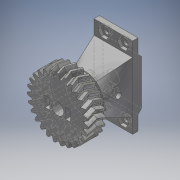
# Autodesk Inventor part: Swivel Joint Driven
Saved by Autodesk Inventor 2019 (Build 230136000, 136)
## iProperties
Created: 2020-04-05
Part Number: Swivel Joint Driven
Material: Steel
Document SubType Name: Modeling
Designer: isaac
Categories: <?xml version="1.0" encoding="UTF-16"?> <MemberInstance><Categories><FamilyTemplate><FamilyTemplateParameter ValueType="xs:double" Id="1" ObjectReferenceKey="da_z" ObjectType="kUserParameterObject"/><FamilyTemplateParameter ValueType="xs:double" Id="2" ObjectReferenceKey="da_b" ObjectType="kUserParameterObject"/><FamilyTemplateParameter ValueType="xs:double" Id="3" ObjectReferenceKey="da_beta" ObjectType="kUserParameterObject"/><FamilyTemplateParameter ValueType="xs:double" Id="4" ObjectReferenceKey="da_da" ObjectType="kUserParameterObject"/><FamilyTemplateParameter ValueType="xs:double" Id="5" ObjectReferenceKey="da_aw" ObjectType="kUserParameterObject"/><FamilyTemplateParameter ValueType="xs:string" Id="6" ObjectReferenceKey="EAIAABAAAACIAQAAAAAAAIAAAAAAAAAA" ObjectType="83910656" SubObjectId="SurfaceGeometry"/></FamilyTemplate><ParamToTemplateMap><ParamToTemplate CategoryParameter="//CategoryParameter[@InternalName='046C89C9-8512-4d59-83FE-43B91F4F132A']" TemplateParameter="1"/><ParamToTemplate CategoryParameter="//CategoryParameter[@InternalName='2552DF32-E462-4b46-AEBF-C6C7768E72AC']" TemplateParameter="2"/><ParamToTemplate CategoryParameter="//CategoryParameter[@InternalName='C9EE641D-15FC-4fae-A226-E94C4372FDD7']" TemplateParameter="3"/><ParamToTemplate><ParamToTemplate CategoryParameter="//CategoryParameter[@InternalName='00B6519A-459B-49c7-AD84-2E56D39A5744']" ConstantValue="-0.025524"/></ParamToTemplate><ParamToTemplate><ParamToTemplate CategoryParameter="//CategoryParameter[@InternalName='04B31F0E-C7A6-4894-AA32-9629BEFACF47']" ConstantValue="1.000000"/></ParamToTemplate><ParamToTemplate><ParamToTemplate CategoryParameter="//CategoryParameter[@InternalName='43CBEC2E-7847-49e7-A936-2F7889FCB2D9']" ConstantValue="0.250000"/></ParamToTemplate><ParamToTemplate><ParamToTemplate CategoryParameter="//CategoryParameter[@InternalName='B1EFC894-105D-4ebd-86BF-FA20ED196853']" ConstantValue="0.333500"/></ParamToTemplate><ParamToTemplate><ParamToTemplate CategoryParameter="//CategoryParameter[@InternalName='51175063-3D10-4879-93E8-6246FE8B403D']" ConstantValue="2060000000.000000"/></ParamToTemplate><ParamToTemplate><ParamToTemplate CategoryParameter="//CategoryParameter[@InternalName='A3A52E27-4454-46a9-B0BD-C932399B70AF']" ConstantValue="0.300000"/></ParamToTemplate><ParamToTemplate><ParamToTemplate CategoryParameter="//CategoryParameter[@InternalName='91B76062-C214-41d9-B1B9-14D2AB99603D']" ConstantValue="0.112500"/></ParamToTemplate><ParamToTemplate><ParamToTemplate CategoryParameter="//CategoryParameter[@InternalName='374E806E-8B8A-4dda-A9AA-1039D6500AD2']" ConstantValue="8.888889"/></ParamToTemplate><ParamToTemplate><ParamToTemplate CategoryParameter="//CategoryParameter[@InternalName='2D373A89-B862-43d6-8D0B-0CBF12AB9F6C']" ConstantValue="0.349066"/></ParamToTemplate><ParamToTemplate CategoryParameter="//CategoryParameter[@InternalName='37777632-D6A2-4fac-9D53-DB8ACD95C989']" TemplateParameter="4"/><ParamToTemplate CategoryParameter="//CategoryParameter[@InternalName='FD1017F1-B727-4f7e-9707-0F86F1FF9423']" TemplateParameter="5"/><ParamToTemplate><ParamToTemplate CategoryParameter="//CategoryParameter[@InternalName='9E1B4470-B2D3-4ff1-B813-535BB4CDF51A']" ConstantValue="3520000.000000"/></ParamToTemplate><ParamToTemplate><ParamToTemplate CategoryParameter="//CategoryParameter[@InternalName='F8452263-BFF6-458c-9FB1-07C4B99E95CD']" ConstantValue="11400000.000000"/></ParamToTemplate><ParamToTemplate><ParamToTemplate CategoryParameter="//CategoryParameter[@InternalName='3E3BB259-FD49-497f-8171-6EBC954A3479']" ConstantValue="2.000000"/></ParamToTemplate><ParamToTemplate CategoryParameter="//CategoryParameter[@InternalName='27C3BAF2-7550-4e4b-AE2C-0DB134B7D9B7']" TemplateParameter="6"/></ParamToTemplateMap><Category DisplayName="Gear" InternalName="DC85795E-93AB-48d5-8EEE-5A27447B64BD" Mnemonic="Gear"><CategoryParameter DisplayName="z" InternalName="046C89C9-8512-4d59-83FE-43B91F4F132A" Mnemonic="z"/><CategoryParameter DisplayName="b" InternalName="2552DF32-E462-4b46-AEBF-C6C7768E72AC" Mnemonic="b"/><CategoryParameter DisplayName="||b|" InternalName="C9EE641D-15FC-4fae-A226-E94C4372FDD7" Mnemonic="beta"/><CategoryParameter DisplayName="x" InternalName="00B6519A-459B-49c7-AD84-2E56D39A5744" Mnemonic="x"/><CategoryParameter DisplayName="a*" InternalName="04B31F0E-C7A6-4894-AA32-9629BEFACF47" Mnemonic="a"/><CategoryParameter DisplayName="c*" InternalName="43CBEC2E-7847-49e7-A936-2F7889FCB2D9" Mnemonic="c"/><CategoryParameter DisplayName="r|.f|*" InternalName="B1EFC894-105D-4ebd-86BF-FA20ED196853" Mnemonic="rf"/><CategoryParameter DisplayName="E" InternalName="51175063-3D10-4879-93E8-6246FE8B403D" Mnemonic="E"/><CategoryParameter DisplayName="||m|" InternalName="A3A52E27-4454-46a9-B0BD-C932399B70AF" Mnemonic="mi"/><Category DisplayName="SpurGear" InternalName="26C5A22E-A91E-4dfd-A3B3-23CCAFAE1764" Mnemonic="SpurGear"><CategoryParameter DisplayName="m" InternalName="91B76062-C214-41d9-B1B9-14D2AB99603D" Mnemonic="m"/><CategoryParameter DisplayName="P" InternalName="374E806E-8B8A-4dda-A9AA-1039D6500AD2" Mnemonic="PP"/><CategoryParameter DisplayName="||a|" InternalName="2D373A89-B862-43d6-8D0B-0CBF12AB9F6C" Mnemonic="alpha"/><CategoryParameter DisplayName="d|.a|" InternalName="37777632-D6A2-4fac-9D53-DB8ACD95C989" Mnemonic="da"/><CategoryParameter DisplayName="a|.w|" InternalName="FD1017F1-B727-4f7e-9707-0F86F1FF9423" Mnemonic="aw"/><CategoryParameter DisplayName="||s||.Flim|" InternalName="9E1B4470-B2D3-4ff1-B813-535BB4CDF51A" Mnemonic="sFlim"/><CategoryParameter DisplayName="||s||.Hlim|" InternalName="F8452263-BFF6-458c-9FB1-07C4B99E95CD" Mnemonic="sHlim"/><CategoryParameter DisplayName="type" InternalName="3E3BB259-FD49-497f-8171-6EBC954A3479" Mnemonic="type"/><CategoryParameter DisplayName="PitchDiameter" InternalName="27C3BAF2-7550-4e4b-AE2C-0DB134B7D9B7" Mnemonic="IDS_PITCHDIAM"/></Category></Category></Categories></MemberInstance>
Density: 1 g/cm^3
Appearance: Steel
CustomPartVersion: 1
Author: isaac
Autodesk Inventor part; units mm, degrees
ref_plane "XY Plane" through (0, 0, 0) normal (0, 0, 1) x (1, 0, 0)
sketch "Sketch1" plane through (0, 0, 0) normal (0, 0, 1) x (1, 0, 0)
  circle A0 centre (0, 0) radius 17.065
  dimension "d0" = 34.13
  constraints: 1 centre point
  measures "d0" diameter of A0
extrude "Extrusion1" add sketch "Sketch1" along normal blind 5
ref_plane "Work Plane2" through (0, 0, 2.5) normal (0, 0, 1) x (1, 0, 0)
sketch "Sketch2" plane through (0, 0, 0) normal (0, 0, -1) x (-1, 0, 0)
  circle A0 centre (0, 0) radius 17.065 projected
  circle A1 centre (0, 0) radius 15.9402
  dimension "d3" = 31.8804
  constraints: 1 centre point, 1 coincident
  measures "d3" diameter of A1
surface extrude "Pitch Diameter" sketch "Sketch2" against normal through all shown no curves A1
ref_plane "Work Plane8" through (0, 0, 0) normal (0.9932384, 0.1160929, 0) x (0, 0, 1)
ref_plane "Work Plane9" through (0, 0, 0) normal (1, 0, 0) x (0, 1, 0)
spur gear teeth "Spur Gear" teeth 27 pitch diameter 31.9382 tip diameter 34.13 root diameter 29.0682 face width 5 helix angle 18 hand right start plane through (0, 0, 0) normal (0, 0, -1) x (-1, 0, 0)
mirror "Mirror1" about plane through (0, 0, 5) normal (0, 0, 1) of "Extrusion1", "Spur Gear"
ref_plane "Work Plane11" through (0, 0, -5) normal (0, 0, -1) x (-1, 0, 0)
sketch "Sketch6" plane through (0, 0, -5) normal (0, 0, -1) x (-1, 0, 0)
  circle A0 centre (0, 0) radius 14.5
  dimension "d52" = 29
  constraints: 1 centre point, 1 coincident
  measures "d52" diameter of A0
extrude "Extrusion2" add sketch "Sketch6" against normal up to surface (5 mm away)
sketch "Sketch7" plane through (0, 0, -5) normal (0, 0, -1) x (-1, 0, 0)
  circle A0 centre (0, 0) radius 10
  dimension "d55" = 20
  constraints: 1 centre point, 1 coincident
  measures "d55" diameter of A0
extrude "Extrusion3" add sketch "Sketch7" along normal blind 15
chamfer "Chamfer1" distance 3.75 angle 45 1 edges at (14.5, 0, -5)
sketch "Sketch9" plane through (-7.9067, 13.688, 10) normal (0, 0, 1) x (0.9546771, 0.2976435, 0)
  point P0 (3.4742, -15.421)
  point P1 (3.4742, -15.421)
  constraints: 1 coincident
hole "Hole1" at (0, 0, 10) direction (0, 0, -1) diameter 7.5 depth 15 tip angle 118
sketch "Sketch10" plane through (0, 0, -20) normal (0, 0, -1) x (-1, 0, 0)
  point P0 (0, 0)
  point P1 (0, 0)
  constraints: 1 coincident
hole "Hole2" at (0, 0, -20) direction (0, 0, 1) diameter 6.5 depth 15
sketch "Sketch11" plane through (0, 0, -20) normal (0, 0, -1) x (-1, 0, 0)
  circle A0 centre (0, 0) radius 3.25 projected
  line L0 (0, 0) -> (-10, 0)
  line L1 (-10, 0) -> (-10, 1)
  line L2 (-10, 1) -> (0, 1)
  line L3 (0, 1) -> (0, 0)
  dimension "d75" = 10
  dimension "d76" = 1
  constraints: 8 end point, 2 parallel, 1 horizontal, 1 perpendicular
  measures "d75" distance of L1.end L2.end
  measures "d76" distance of L0.end L1.end
extrude "Extrusion4" cut sketch "Sketch11" against normal up to surface (15 mm away) contours L2 L3 L0 A0 | A0 L0 L1 L2 picked at (-1.0308, 0.6667)
ref_plane "Work Plane13" through (10, 0, 0) normal (1, 0, 0) x (0, 1, 0)
sketch "Sketch12" plane through (10, 0, 0) normal (1, 0, 0) x (0, 1, 0)
  line L0 (10, -5) -> (10, -20) projected
  line L1 (0, -5) -> (10, -5)
  line L2 (10, -5) -> (10, -6)
  line L3 (10, -6) -> (0, -6)
  line L4 (0, -6) -> (0, -5)
  point P0 (0, 0)
  dimension "d80" = 1
  constraints: 8 end point, 2 parallel, 1 horizontal, 1 perpendicular, 1 point on line
  measures "d80" distance of L1.end L2.end
extrude "Extrusion5" cut sketch "Sketch12" against normal blind 20
ref_plane "Work Plane14" through (0, 10, 0) normal (0, 1, 0) x (-1, 0, 0)
sketch "Sketch13" plane through (0, 10, 0) normal (0, 1, 0) x (-1, 0, 0)
  line L0 (-10, -5) -> (-10, -20) construction
  line L1 (-10, -20) -> (10, -20) construction
  line L2 (-10, -5) -> (-6.5, -5) construction
  line L3 (-6.5, -5) -> (-6.5, -20) construction
  line L4 (-6.5, -20) -> (-10, -20) construction
  line L5 (-10, -20) -> (-10, -5) construction
  point P0 (0, 0)
  point P1 (-9.9499, -20)
  point P2 (-6.5, -12.5)
  dimension "d84" = 3.5
  constraints: 8 end point, 2 parallel, 1 horizontal, 1 midpoint, 1 perpendicular, 1 point on line
  measures "d84" distance of L3.end L4.end
hole "Hole3" at (6.5, 10, -12.5) direction (0, -1, 0) diameter 3.5 depth 9 counterbore diameter 6 counterbore depth 7
ref_plane "Work Plane15" through (0, -10, 0) normal (0, 1, 0) x (-1, 0, 0)
sketch "Sketch14" plane through (0, -10, 0) normal (0, 1, 0) x (-1, 0, 0)
  circle A0 centre (-6.5, -12.5) radius 1.75 projected
  point P0 (0, 0)
  constraints: 1 coincident
hole "Hole4" at (6.5, -10, -12.5) direction (0, 1, 0) diameter 3.5 depth 10
sketch "Sketch15" plane through (0, -10, 0) normal (0, 1, 0) x (-1, 0, 0)
  circle A0 centre (-6.5, -12.5) radius 3 projected
  line L0 (-6.5, -15.6754) -> (-9.25, -14.0877)
  line L1 (-9.25, -14.0877) -> (-9.25, -10.9123)
  line L2 (-9.25, -10.9123) -> (-6.5, -9.3246)
  line L3 (-6.5, -9.3246) -> (-3.75, -10.9123)
  line L4 (-3.75, -10.9123) -> (-3.75, -14.0877)
  line L5 (-3.75, -14.0877) -> (-6.5, -15.6754)
  point P0 (0, 0)
  dimension "d100" = 5.5
  constraints: 12 end point, 1 coincident, 13 other
  measures "d100" distance between parallel lines of L4 L1
extrude "Extrusion6" cut sketch "Sketch15" along normal blind 8 contours L4 A0 L5 L0 L1 L2 L3 | A0 L3 L4 | L4 L5 A0 | A0 L2 L3 | L5 L0 A0 | A0 L1 L2 | L0 L1 A0
sketch "Sketch16" plane through (0, 0, -20) normal (0, 0, -1) x (-1, 0, 0)
  arc A0 (-3.25, 0) -> (3.25, 0) centre (0, 0) ccw projected
  arc A1 (-3.25, 0) -> (3.25, 0) centre (0, 0) ccw
  line L0 (-10, 0) -> (-3.75, 0) projected
  arc A2 (-10, 0) -> (-9.9499, 1) centre (0, 0) ccw projected
  arc A3 (-10, 0) -> (10, 0) centre (0, 0) ccw
  line L1 (-3.25, 0) -> (-10, 0) projected
  line L2 (-10, 0) -> (-3.25, 0)
  line L3 (3.25, 0) -> (10, 0) projected
  line L4 (3.25, 0) -> (10, 0)
  constraints: 5 point on circle, 4 end point, 2 centre point, 2 coincident, 1 collinear, 1 horizontal
extrude "Extrusion7" add sketch "Sketch16" along normal blind 1
chamfer "Chamfer2" distance 0.75 angle 45 1 edges at (0, -10, -5)
sketch "Sketch18" plane through (0, 0, -21) normal (0, 0, -1) x (-1, 0, 0)
  line L0 (-10.75, 22.55) -> (10.75, 22.55)
  line L1 (10.75, 22.55) -> (10.75, -22.55)
  line L2 (10.75, -22.55) -> (-10.75, -22.55)
  line L3 (-10.75, -22.55) -> (-10.75, 22.55)
  line L4 (-10.75, 22.55) -> (10.75, -22.55) construction
  line L5 (10.75, 22.55) -> (-10.75, -22.55) construction
  point P0 (0, 0)
  dimension "d116" = 21.5
  dimension "d117" = 45.1
  constraints: 12 end point, 2 midpoint, 2 parallel, 1 horizontal, 1 perpendicular
  measures "d116" distance of L1.end L2.end
  measures "d117" distance of L0.end L1.end
extrude "Extrusion9" add sketch "Sketch18" along normal blind 5
sketch "Sketch19" plane through (0, 0, -26) normal (0, 0, -1) x (-1, 0, 0)
  line L0 (-10.75, -22.55) -> (-10.75, 22.55) projected
  line L1 (10.75, 22.55) -> (10.75, -22.55) projected
  line L2 (-10.75, 22.55) -> (10.75, 22.55)
  line L3 (10.75, 22.55) -> (10.75, 12.55)
  line L4 (10.75, 12.55) -> (-10.75, 12.55)
  line L5 (-10.75, 12.55) -> (-10.75, 22.55)
  line L6 (-10.75, -22.55) -> (10.75, -22.55)
  line L7 (10.75, -22.55) -> (10.75, -12.55)
  line L8 (10.75, -12.55) -> (-10.75, -12.55)
  line L9 (-10.75, -12.55) -> (-10.75, -22.55)
  point P0 (0, 0)
  dimension "d120" = 10
  dimension "d121" = 10
  constraints: 16 end point, 4 parallel, 2 horizontal, 2 perpendicular, 2 point on line
  measures "d120" distance of L2.end L3.end
  measures "d121" distance of L7.end L6.end
extrude "Extrusion10" cut sketch "Sketch19" against normal blind 2 contours L0 L8 L1 L6 | L0 L2 L1 L4
chamfer "Chamfer4" distance 2 angle 45 2 edges at (0, 12.55, -24) (0, -12.55, -24)
sketch "Sketch20" plane through (-7.9067, 13.688, 10) normal (0, 0, 1) x (0.9546771, 0.2976435, 0)
  circle A0 centre (3.4742, -15.421) radius 3.75
  circle A1 centre (3.4742, -15.421) radius 3.75 projected
  circle A2 centre (3.4742, -15.421) radius 3.25
  constraints: 2 centre point, 2 coincident
extrude "Extrusion11" add sketch "Sketch20" against normal up to surface round surface about axis through (0, 0, -6.1266) along (0, 0, 1) radius 1.875 half angle 59 far side no
sketch "Sketch21" plane through (0, 0, -21) normal (0, 0, 1) x (1, 0, 0)
  line L0 (10.75, 22.55) -> (-10.75, 22.55) construction
  line L1 (10.75, 14.55) -> (10.75, 12.55) construction
  line L2 (-10.75, 22.55) -> (10.75, 22.55) construction
  line L3 (10.75, 22.55) -> (10.75, 14.55) construction
  line L4 (10.75, 14.55) -> (-10.75, 14.55) construction
  line L5 (-10.75, 14.55) -> (-10.75, 22.55) construction
  line L6 (-10.75, 14.55) -> (10.75, 14.55) construction
  line L7 (-10.75, 22.55) -> (10.75, 14.55) construction
  line L8 (10.75, 22.55) -> (-10.75, 14.55) construction
  line L9 (0, 18.55) -> (10.75, 18.55) construction
  line L10 (0, 18.55) -> (-10.75, 18.55) construction
  line L11 (-10.75, 22.55) -> (-10.75, -22.55) construction
  point P0 (0, 0)
  point P1 (-10.75, 0)
  point P2 (-5.375, 18.55)
  point P3 (5.375, 18.55)
  constraints: 16 end point, 4 midpoint, 2 parallel, 2 point on line, 1 horizontal, 1 perpendicular
hole "Hole5" at (-5.375, 18.55, -21) at (5.375, 18.55, -21) direction (0, 0, -1) diameter 3.5 depth 3
sketch "Sketch22" plane through (0, 0, -21) normal (0, 0, 1) x (1, 0, 0)
  circle A0 centre (-5.375, 18.55) radius 1.75 projected
  line L0 (-8.5504, 18.55) -> (-6.9627, 21.3)
  line L1 (-6.9627, 21.3) -> (-3.7873, 21.3)
  line L2 (-3.7873, 21.3) -> (-2.1996, 18.55)
  line L3 (-2.1996, 18.55) -> (-3.7873, 15.8)
  line L4 (-3.7873, 15.8) -> (-6.9627, 15.8)
  line L5 (-6.9627, 15.8) -> (-8.5504, 18.55)
  circle A1 centre (5.375, 18.55) radius 1.75 projected
  line L6 (8.5504, 18.55) -> (6.9627, 15.8)
  line L7 (6.9627, 15.8) -> (3.7873, 15.8)
  line L8 (3.7873, 15.8) -> (2.1996, 18.55)
  line L9 (2.1996, 18.55) -> (3.7873, 21.3)
  line L10 (3.7873, 21.3) -> (6.9627, 21.3)
  line L11 (6.9627, 21.3) -> (8.5504, 18.55)
  point P0 (0, 0)
  dimension "d139" = 5.5
  dimension "d140" = 5.5
  constraints: 24 end point, 2 coincident, 26 other
  measures "d139" distance between parallel lines of L4 L1
  measures "d140" distance between parallel lines of L7 L10
extrude "Extrusion12" cut sketch "Sketch22" against normal blind 1.75
mirror "Mirror2" about plane through (0, 0, 0) normal (0, 1, 0) of "Hole5", "Extrusion12"
ref_plane "Work Plane16" through (10, 0, 0) normal (1, 0, 0) x (0, 1, 0)
sketch "Sketch23" plane through (10, 0, 0) normal (1, 0, 0) x (0, 1, 0)
  line L0 (3.25, -6) -> (0, -6) projected
  line L1 (0, -20) -> (10, -20) projected
  line L2 (0, -6) -> (10, -6)
  line L3 (10, -6) -> (10, -20)
  line L4 (10, -20) -> (0, -20)
  line L5 (0, -20) -> (0, -6)
  point P0 (0, 0)
  point P1 (1, -6)
  point P2 (1, -20)
  constraints: 8 end point, 2 parallel, 1 horizontal, 1 perpendicular
extrude "Extrusion13" cut sketch "Sketch23" against normal up to next
mirror "Mirror3" about plane through (0, 0, 0) normal (1, 0, 0) of "Extrusion6", "Hole4"
chamfer "Chamfer6" distance 4.5 angle 45 1 edges at (0, -10, -21)
sketch "Sketch24" plane through (-10.75, 0, -21) normal (-1, 0, 0) x (0, 0, 1)
  line L0 (0, -22.55) -> (-3, -22.55) projected
  line L1 (16, 0) -> (16, 10.75) projected
  line L2 (0, -22.55) -> (16, -22.55)
  line L3 (16, -22.55) -> (16, 10.75)
  line L4 (16, 10.75) -> (0, 10.75)
  line L5 (0, 10.75) -> (0, -22.55)
  point P0 (21, 0)
  constraints: 8 end point, 2 parallel, 1 horizontal, 1 perpendicular
extrude "Extrusion14" cut sketch "Sketch24" against normal through all
sketch "Sketch26" plane through (0, 0, -21) normal (0, 0, 1) x (1, 0, 0)
  line L0 (10.75, 14.55) -> (10.75, 22.55) projected
  line L1 (-10.75, -14.55) -> (10.75, -14.55)
  line L2 (10.75, -14.55) -> (10.75, 14.55)
  line L3 (10.75, 14.55) -> (-10.75, 14.55)
  line L4 (-10.75, 14.55) -> (-10.75, -14.55)
  line L5 (-10.75, -14.55) -> (10.75, 14.55) construction
  line L6 (10.75, -14.55) -> (-10.75, 14.55) construction
  point P0 (0, 0)
  dimension "d151" = 21.5
  constraints: 12 end point, 2 midpoint, 2 parallel, 1 horizontal, 1 perpendicular
  measures "d151" distance of L3.end L0.start
loft "Loft1" add profiles "Sketch26" section 2 edges at (10.75, 0, -5)
sketch "Sketch27" plane through (-7.9067, 13.688, 10) normal (0, 0, 1) x (0.9546771, 0.2976435, 0)
  circle A0 centre (3.4742, -15.421) radius 3.325
  dimension "d156" = 6.65
  constraints: 1 centre point, 1 coincident
  measures "d156" diameter of A0
extrude "Extrusion15" cut sketch "Sketch27" against normal blind 31
ref_plane "Work Plane17" through (-5.75, 22.55, -24) normal (-1, 0, 0) x (0, 0, 1)
sketch "Sketch28" plane through (-5.75, 22.55, -24) normal (-1, 0, 0) x (0, 0, 1)
  line L0 (34, -25.875) -> (3, -25.875) construction
  line L1 (34, -19.225) -> (3, -19.225) construction
  line L2 (18.5, -25.875) -> (3, -25.875) construction
  line L3 (3, -25.875) -> (3, -19.225) construction
  line L4 (3, -19.225) -> (18.5, -19.225) construction
  line L5 (18.5, -19.225) -> (18.5, -25.875) construction
  line L6 (3, -19.225) -> (3, -25.875) construction
  line L7 (3, -22.55) -> (18.5, -22.55) construction
  line L8 (7.3436, -22.55) -> (9.0468, -19.6)
  line L9 (9.0468, -19.6) -> (12.4532, -19.6)
  line L10 (12.4532, -25.5) -> (9.0468, -25.5)
  line L11 (9.0468, -25.5) -> (7.3436, -22.55)
  line L12 (12.4532, -25.5) -> (34, -25.5)
  line L13 (34, -25.5) -> (34, -19.6)
  line L14 (34, -19.6) -> (12.4532, -19.6)
  line L15 (9.0468, -25.5) -> (34, -25.5)
  line L16 (34, -25.5) -> (34, -19.6)
  line L17 (34, -19.225) -> (34, -25.875) projected
  line L18 (34, -19.6) -> (9.0468, -19.6)
  line L19 (9.0468, -19.6) -> (7.3436, -22.55)
  line L20 (7.3436, -22.55) -> (9.0468, -25.5)
  point P0 (24, -22.55)
  point P1 (10.75, -22.55)
  dimension "d160" = 5.9
  constraints: 34 end point, 5 collinear, 4 midpoint, 3 parallel, 2 horizontal, 2 perpendicular, 2 point on line, 8 other
  measures "d160" distance between parallel lines of L9 L10
extrude "Extrusion16" cut sketch "Sketch28" along normal mid plane 2.7
sketch "Sketch29" plane through (-10.75, 22.55, -24) normal (-1, 0, 0) x (0, 0, 1)
  circle A0 centre (10.75, -22.55) radius 2.95 construction
  point P0 (24, -22.55)
  constraints: 1 centre point, 1 coincident
hole "Hole6" at (-10.75, 0, -13.25) direction (1, 0, 0) diameter 3.1 depth 10
mirror "Mirror4" about plane through (0, 0, 0) normal (1, 0, 0) of "Extrusion16", "Hole6"
equation "\"d0\" = da_da"
equation "\"d1\" = da_b"
equation "\"d3\" = da_dw"
equation "\"d16\" = da_aw"
equation "\"d43\" = da_aw"
equation "\"d46\" = da_aw"
equation "\"da_da\" = 34.130032"
equation "\"da_b\" = 5"
equation "\"da_dw\" = 31.880377"
equation "\"da_aw\" = 31.29"
body "Solid1"
body "Srf1"
